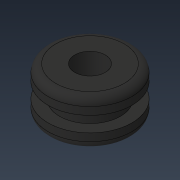
# Autodesk Inventor part: Gummitülle 3mm
Saved by Autodesk Inventor 2022.1 (Build 261234020, 234B)
## iProperties
Part Number: Gummitülle 3mm
Material: Gummi
Document SubType Name: Modeling
Designer: rYan
Mass: 0.181866 g
Surface Area: 3.07339 cm^2
Volume: 0.195554 cm^3
Density: 0.93 g/cm^3
Appearance: Gummi - Schwarz
Author: rYan
Title: 1722-1291-ND
Autodesk Inventor part; units mm, degrees
ref_plane "YZ Plane" through (0, 0, 0) normal (1, 0, 0) x (0, 1, 0)
ref_plane "XZ Plane" through (0, 0, 0) normal (0, 1, 0) x (-1, 0, 0)
ref_plane "XY Plane" through (0, 0, 0) normal (0, 0, 1) x (1, 0, 0)
sketch "Skizze2" plane through (0, 0, 0) normal (0, 1, 0) x (-1, 0, 0)
  line L0 (-1.5875, -2.3813) -> (-1.5875, 2.3812)
  line L1 (-1.5875, 2.3812) -> (-3.5719, 2.3812)
  arc A0 (-3.5719, 2.3812) -> (-4.3656, 1.5875) centre (-3.5719, 1.5875) ccw
  line L2 (-4.3656, 1.5875) -> (-4.3656, 0.7937)
  line L3 (-4.3656, 0.7937) -> (-3.175, 0.7937)
  line L4 (-3.175, 0.7937) -> (-3.175, -0.7937)
  line L5 (-3.175, -0.7937) -> (-4.3656, -0.7937)
  line L6 (-4.3656, -0.7937) -> (-4.3656, -1.5875)
  line L7 (-1.5875, -2.3813) -> (-3.5719, -2.3813)
  arc A1 (-4.3656, -1.5875) -> (-3.5719, -2.3813) centre (-3.5719, -1.5875) ccw
  line L8 (0, 2.3813) -> (0, -2.3813)
  line L9 (-5.436, 0) -> (0.906, 0) projected
  point P0 (0, 0)
  point P1 (0, 0)
  dimension "d0" = 3.175
  dimension "d1" = 6.35
  dimension "d2" = 8.7312
  dimension "d3" = 1.5875
  dimension "d4" = 4.7625
  dimension "d5" = 0.7937
  constraints: 18 end point, 4 perpendicular, 4 point on circle, 4 point on line, 4 tangent, 3 vertical, 2 centre point, 1 coincident, 1 horizontal, 1 midpoint, 2 other
  measures "d0" diameter of L0 L8
  measures "d1" diameter of L4 L8
  measures "d2" diameter of L2 L8
  measures "d3" distance between parallel lines of L3 L5
  measures "d4" distance between parallel lines of L1 L7
  measures "d5" radius of A0
revolve "Umdrehung1" add sketch "Skizze2" angle 360 about axis through (0, 0, 2.3813) along (0, 0, -1)
